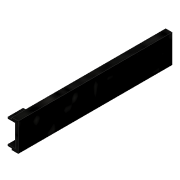
# Autodesk Inventor part: Wire Cover Strengthened
Saved by Autodesk Inventor 2017 (Build 210142000, 142)
## iProperties
Created: 2016-08-18
Part Number: Wire Cover Strengthened
Material: Generic
Document SubType Name: Modeling
Designer: ge937963
Density: 1 g/cm^3
Appearance: Smooth - Black
Author: ge937963
Autodesk Inventor part; units mm, degrees
ref_plane "YZ Plane" through (0, 0, 0) normal (1, 0, 0) x (0, 1, 0)
sketch "Sketch1" plane through (0, 0, 0) normal (0, 0, 1) x (1, 0, 0)
  arc A0 (-8.0491, 3.1697) -> (-8.0491, -3.1803) centre (-17.5665, -0.0053) ccw projected
  line L0 (-1.651, -3.1803) -> (-8.0491, -3.1803) projected
  line L1 (-1.651, -5.461) -> (-1.651, -3.1803) projected
  line L2 (0, -5.461) -> (-1.651, -5.461) projected
  line L3 (0, -5.461) -> (0, -6.35) projected
  line L4 (3.175, -6.35) -> (0, -6.35) projected
  line L5 (3.175, 6.35) -> (3.175, -6.35) projected
  line L6 (3.175, 6.35) -> (0, 6.35) projected
  line L7 (0, 6.35) -> (0, 5.461) projected
  line L8 (-1.651, 5.461) -> (0, 5.461) projected
  line L9 (-1.651, 3.1697) -> (-1.651, 5.461) projected
  line L10 (-1.651, 3.1697) -> (-8.0491, 3.1697) projected
  line L11 (3.175, 5.842) -> (0.508, 5.842)
  line L12 (0.508, 5.842) -> (0.508, -5.842)
  line L13 (0.508, -5.842) -> (3.175, -5.842)
  line L14 (3.175, -5.842) -> (3.175, 5.842)
  line L15 (0.508, 5.207) -> (1.651, 5.207)
  line L16 (1.651, 5.207) -> (1.651, -5.207)
  line L17 (1.651, -5.207) -> (0.508, -5.207)
  line L18 (0.508, -5.207) -> (0.508, 5.207)
  point P0 (0, 0)
  dimension "d0" = 0.508
  dimension "d1" = 0.508
  dimension "d2" = 0.508
  dimension "d3" = 0.635
  dimension "d4" = 0.635
  dimension "d5" = 1.524
  constraints: 16 end point, 4 parallel, 2 horizontal, 2 perpendicular, 2 point on line
  measures "d0" distance between parallel lines of L6 L11
  measures "d1" distance between parallel lines of L4 L13
  measures "d2" distance between parallel lines of L7 L12
  measures "d3" distance between parallel lines of L11 L15
  measures "d4" distance between parallel lines of L13 L17
  measures "d5" distance between parallel lines of L5 L16
ref_plane "Work Plane1" through (0, -6.35, 57.7672) normal (0, 0, -1) x (0, 1, 0)
extrude "Extrusion1" add sketch "Sketch1" along normal up to surface (57.7672 mm away) contours L5 L13 L12 L17 L16 L15 L11
ref_plane "Work Plane2" through (2.413, 0, 64.1172) normal (0, 0, -1) x (-1, 0, 0)
sketch "Sketch2" plane through (2.413, 0, 64.1172) normal (0, 0, -1) x (-1, 0, 0)
  line L0 (-0.762, -5.842) -> (-0.762, 5.842) projected
  line L1 (-0.762, 5.08) -> (3.556, 5.08)
  line L2 (3.556, 5.08) -> (3.556, 4.572)
  line L3 (3.556, 4.572) -> (-0.762, 4.572)
  line L4 (-0.762, 4.572) -> (-0.762, 5.08)
  line L5 (-0.762, -5.08) -> (3.556, -5.08)
  line L6 (3.556, -5.08) -> (3.556, -4.572)
  line L7 (3.556, -4.572) -> (-0.762, -4.572)
  line L8 (-0.762, -4.572) -> (-0.762, -5.08)
  line L9 (1.905, -5.207) -> (0.762, -5.207) projected
  line L10 (0.762, 5.207) -> (1.905, 5.207) projected
  line L11 (-0.762, 5.08) -> (0.508, 5.08)
  line L12 (0.508, 5.08) -> (0.508, -5.08)
  line L13 (0.508, -5.08) -> (-0.762, -5.08)
  line L14 (-0.762, -5.08) -> (-0.762, 5.08)
  point P0 (2.413, 0)
  dimension "d8" = 0.508
  dimension "d9" = 4.318
  dimension "d10" = 4.318
  dimension "d11" = 0.508
  dimension "d12" = 0.127
  dimension "d13" = 0.127
  constraints: 24 end point, 6 parallel, 3 horizontal, 3 perpendicular, 3 point on line
  measures "d8" distance of L1.end L2.end
  measures "d9" distance between parallel lines of L0 L2
  measures "d10" distance of L7.end L6.end
  measures "d11" distance of L5.end L6.end
  measures "d12" distance between parallel lines of L9 L5
  measures "d13" distance between parallel lines of L10 L1
extrude "Extrusion2" add sketch "Sketch2" along normal up to surface (6.35 mm away)
sketch "Sketch3" plane through (1.651, -5.207, 0) normal (-1, 0, 0) x (0, 0, 1)
  line L0 (0, 10.414) -> (57.7672, 10.414) projected
  line L1 (57.7672, 10.414) -> (56.4972, 10.414)
  line L2 (56.4972, 10.414) -> (56.4972, 9.779)
  line L3 (56.4972, 9.779) -> (57.7672, 9.779)
  line L4 (57.7672, 9.779) -> (57.7672, 10.414)
  line L5 (57.7672, -0.635) -> (57.7672, 0.127) projected
  line L6 (57.7672, 0) -> (56.4972, 0)
  line L7 (56.4972, 0.635) -> (57.7672, 0.635)
  line L8 (57.7672, 0.635) -> (57.7672, 0)
  line L9 (64.1172, 9.779) -> (57.7672, 9.779) projected
  line L10 (56.4972, 0.635) -> (56.4972, 0)
  point P0 (0, 5.207)
  dimension "d16" = 1.27
  constraints: 16 end point, 4 parallel, 2 horizontal, 2 perpendicular, 2 point on line, 1 coincident, 1 horizontal alignment
  measures "d16" distance between parallel lines of L4 L2
extrude "Extrusion3" add sketch "Sketch3" along normal up to surface (1.143 mm away)
sketch "Sketch4" plane through (3.175, -5.842, 0) normal (1, 0, 0) x (0, 0, -1)
  line L0 (0, 11.684) -> (-57.7672, 11.684) projected
  line L1 (0.0018, 0) -> (-0.5062, 0)
  line L2 (-0.5062, 0) -> (-0.5062, 11.684)
  line L3 (-0.5062, 11.684) -> (0.0018, 11.684)
  line L4 (0.0018, 11.684) -> (0.0018, 0)
  point P0 (0, 5.842)
  dimension "d19" = 0.508
  constraints: 8 end point, 2 parallel, 1 horizontal, 1 perpendicular, 1 point on line
  measures "d19" distance of L1.start L1.end
extrude "Extrusion4" cut sketch "Sketch4" against normal blind 25.4
sketch "Sketch5" plane through (3.175, -5.08, 64.1172) normal (1, 0, 0) x (0, 0, -1)
  line L0 (63.611, -0.762) -> (63.611, 10.922) projected
  line L1 (63.611, 10.922) -> (6.35, 10.922) projected
  line L2 (6.35, 10.16) -> (6.35, 10.922) projected
  line L3 (0, 10.16) -> (6.35, 10.16) projected
  line L4 (0, 10.16) -> (0, 0) projected
  line L5 (0, 0) -> (6.35, 0) projected
  line L6 (6.35, -0.762) -> (6.35, 0) projected
  line L7 (63.611, -0.762) -> (6.35, -0.762) projected
  line L8 (6.35, 10.16) -> (6.35, 10.922) projected
  line L9 (0, 9.652) -> (0, 10.16) projected
  line L10 (6.35, 10.922) -> (0, 10.922)
  line L11 (0, 10.922) -> (0, 10.16)
  line L12 (0, 10.16) -> (6.35, 10.16)
  line L13 (6.35, 10.16) -> (6.35, 10.922)
  line L14 (0, 10.16) -> (0, 0) projected
  line L15 (6.35, -0.762) -> (6.35, 0) projected
  line L16 (0, 0) -> (6.35, 0)
  line L17 (6.35, 0) -> (6.35, -0.762)
  line L18 (6.35, -0.762) -> (0, -0.762)
  line L19 (0, -0.762) -> (0, 0)
  point P0 (64.1172, 5.08)
  constraints: 16 end point, 4 parallel, 2 horizontal, 2 perpendicular
extrude "Extrusion5" add sketch "Sketch5" against normal up to surface (4.318 mm away) contours L18 L19 L5 L6 | L2 L3 L11 L10
sketch "Sketch6" plane through (2.413, 0, 64.1172) normal (0, 0, 1) x (1, 0, 0)
  line L0 (-0.508, -4.572) -> (-0.508, 4.572) projected
  line L1 (-3.556, -4.572) -> (-0.508, -4.572) projected
  line L2 (-3.556, -4.572) -> (-3.556, -5.842) projected
  line L3 (0.762, -5.842) -> (-3.556, -5.842) projected
  line L4 (0.762, 5.842) -> (0.762, -5.842) projected
  line L5 (0.762, 5.842) -> (-3.556, 5.842) projected
  line L6 (-3.556, 4.572) -> (-3.556, 5.842) projected
  line L7 (-0.508, 4.572) -> (-3.556, 4.572) projected
  line L8 (0.762, -5.842) -> (-3.556, -5.842) projected
  line L9 (-3.556, -5.842) -> (-1.905, -5.842)
  line L10 (-1.905, -5.842) -> (-1.905, -5.207)
  line L11 (-1.905, -5.207) -> (-3.556, -5.207)
  line L12 (-3.556, -5.207) -> (-3.556, -5.842)
  line L13 (-3.556, 5.842) -> (-1.905, 5.842)
  line L14 (-1.905, 5.842) -> (-1.905, 5.207)
  line L15 (-1.905, 5.207) -> (-3.556, 5.207)
  line L16 (-3.556, 5.207) -> (-3.556, 5.842)
  line L17 (-1.905, 5.842) -> (-1.905, 5.207) projected
  line L18 (-1.905, 4.572) -> (-1.905, 5.207) projected
  line L19 (-1.905, 5.842) -> (-1.905, 4.572) projected
  line L20 (-1.905, -5.207) -> (-1.905, -5.842) projected
  line L21 (-1.905, -4.572) -> (-1.905, -5.842) projected
  line L22 (-1.905, -5.207) -> (-1.905, -4.572) projected
  line L23 (-0.762, -5.207) -> (-1.905, -5.207) projected
  line L24 (-1.905, -5.207) -> (-0.762, -5.207) projected
  line L25 (-1.905, 5.207) -> (-0.762, 5.207) projected
  line L26 (-0.762, 5.207) -> (-1.905, 5.207) projected
  point P0 (-2.413, 0)
  constraints: 16 end point, 4 parallel, 2 horizontal, 2 midpoint, 2 perpendicular, 1 point on line
extrude "Extrusion6" cut sketch "Sketch6" against normal blind 25.4 contours L10 L3 L2 L11 | L15 L6 L5 L14
body "Solid1"
